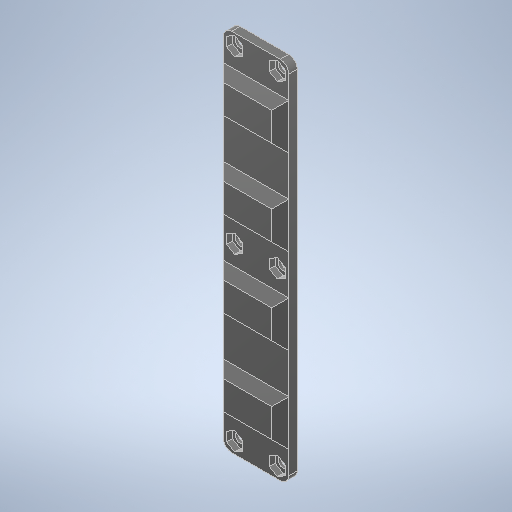
# Autodesk Inventor part: 3D_frame-connect-base2-1
Saved by Autodesk Inventor 2025 (Build 290162000, 162)
## iProperties
Created: 2024-07-30
Part Number: 3D_frame-connect-base2-1
Material: 一般
Document SubType Name: Modeling
Designer: 8326d
Density: 1 g/cm^3
Appearance: 滑らか - 黒
Author: 8326d
## iProperties of the stored document 3D_frame-connect-base2-1_3D プリント.ipt
Created: 2024-08-04
Part Number: 3D_frame-connect-base2-1_3D プリント
Material: 一般
Document SubType Name: Modeling
Designer: 8326d
Density: 1 g/cm^3
Appearance: 既定
Author: 8326d
Autodesk Inventor part; units mm, degrees
ref_plane "YZ Plane" through (0, 0, 0) normal (1, 0, 0) x (0, 1, 0)
ref_plane "XZ Plane" through (0, 0, 0) normal (0, 1, 0) x (-1, 0, 0)
ref_plane "XY Plane" through (0, 0, 0) normal (0, 0, 1) x (1, 0, 0)
sketch "スケッチ1" plane through (0, 0, 0) normal (0, 0, 1) x (1, 0, 0)
  line L0 (-11.5, -64) -> (11.5, -64)
  line L1 (11.5, -64) -> (11.5, 64)
  line L2 (11.5, 64) -> (-11.5, 64)
  line L3 (-11.5, 64) -> (-11.5, -64)
  line L4 (-11.5, -64) -> (11.5, 64) construction
  line L5 (11.5, -64) -> (-11.5, 64) construction
  point P0 (0, 0)
  dimension "d0" = 23
  dimension "d1" = 128
  constraints: 12 end point, 2 midpoint, 2 parallel, 1 horizontal, 1 perpendicular
  measures "d0" distance of L2.end L1.end
  measures "d1" distance of L1.end L0.end
extrude "押し出し1" add sketch "スケッチ1" along normal blind 3
sketch "スケッチ2" plane through (0, 0, 3) normal (0, 0, 1) x (1, 0, 0)
  line L0 (-7.5, -60) -> (7.5, -60) construction
  line L1 (7.5, -60) -> (7.5, 60) construction
  line L2 (7.5, 60) -> (-7.5, 60) construction
  line L3 (-7.5, 60) -> (-7.5, -60) construction
  line L4 (-7.5, -60) -> (7.5, 60) construction
  line L5 (7.5, -60) -> (-7.5, 60) construction
  point P0 (0, 0)
  point P1 (7.5, 0)
  point P2 (-7.5, 0)
  dimension "d4" = 15
  dimension "d5" = 120
  constraints: 12 end point, 4 coincident, 4 midpoint, 2 parallel, 1 horizontal, 1 perpendicular
  measures "d4" distance of L2.end L1.end
  measures "d5" distance of L1.end L0.end
hole "穴1" at (-7.5, 60, 3) at (7.5, 60, 3) at (7.5, 0, 3) at (-7.5, 0, 3) at (-7.5, -60, 3) at (7.5, -60, 3) direction (0, 0, -1) diameter 3.5 end through all
sketch "スケッチ3" plane through (0, 0, 3) normal (0, 0, 1) x (1, 0, 0)
  circle A0 centre (-7.5, 60) radius 1.75 projected
  line L0 (-7.5, 63.2332) -> (-4.7, 61.6166)
  line L1 (-4.7, 61.6166) -> (-4.7, 58.3834)
  line L2 (-4.7, 58.3834) -> (-7.5, 56.7668)
  line L3 (-7.5, 56.7668) -> (-10.3, 58.3834)
  line L4 (-10.3, 58.3834) -> (-10.3, 61.6166)
  line L5 (-10.3, 61.6166) -> (-7.5, 63.2332)
  point P0 (0, 0)
  dimension "d13" = 5.6
  constraints: 12 end point, 1 coincident, 1 vertical alignment, 13 other
  measures "d13" distance between parallel lines of L1 L4
extrude "押し出し2" cut sketch "スケッチ3" against normal blind 2
pattern_linear "矩形状パターン1" count 2 spacing 15 along (1, 0, 0) count 3 spacing 60 along (0, -1, 0) of "押し出し2"
sketch "スケッチ4" plane through (11.5, -64, 0) normal (1, 0, 0) x (0, 0, -1)
  line L0 (-3, 0) -> (-3, 128) projected
  line L1 (-3, 71) -> (-6, 74)
  line L2 (-6, 74) -> (-6, 84)
  line L3 (-6, 84) -> (-3, 87)
  line L4 (0, 0) -> (0, 128) projected
  point P0 (0, 64)
  point P1 (0, 64)
  point P2 (-6, 79)
  dimension "d22" = 45
  dimension "d23" = 45
  dimension "d24" = 10
  dimension "d25" = 3
  dimension "d26" = 15
  constraints: 6 end point, 2 midpoint, 2 point on line, 1 vertical
  measures "d22" angle of L0 L1
  measures "d23" angle of L0 L3
  measures "d24" distance of L1.end L2.end
  measures "d25" distance between parallel lines of L0 L2
  measures "d26" vertical distance of point (0, 64) point (-6, 79)
extrude "押し出し3" add sketch "スケッチ4" against normal up to surface (23 mm away)
pattern_linear "矩形状パターン2" count 4 spacing 30 along (0, -1, 0) of "押し出し3" first direction both ways yes
chamfer "面取り1" distance 3 angle 45 8 edges at (11.5, -45, 6) (-11.5, -45, 6) (-11.5, -15, 6) (11.5, -15, 6) (11.5, 15, 6) (-11.5, 15, 6) (11.5, 45, 6) (-11.5, 45, 6)
fillet "フィレット1" radius 3 4 edges at (-11.5, 64, 1.5) (11.5, 64, 1.5) (-11.5, -64, 1.5) (11.5, -64, 1.5)
equation "\"d23\" = d22"
